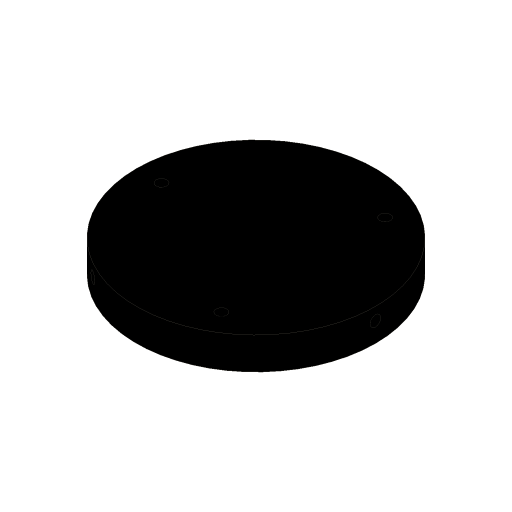
# Autodesk Inventor part: Engine bulkhead
Saved by Autodesk Inventor 2024 (Build 280153000, 153)
## iProperties
Created: 2023-12-30
Part Number: Engine bulkhead
Material: Steel AISI 1006 85 HR
Document SubType Name: Modeling
Designer: Jamie
Density: 7.872 g/cm^3
Appearance: Steel
Mass: 203.39 g
Surface Area: 95.0094 cm^2
Volume: 25.8372 cm^3
Author: Jamie
Autodesk Inventor part; units mm, degrees
ref_plane "XZ Plane" through (0, 0, 0) normal (0, 1, 0) x (-1, 0, 0)
ref_plane "XY Plane" through (0, 0, 0) normal (0, 0, 1) x (1, 0, 0)
sketch "Sketch1" plane through (0, 0, 0) normal (0, 1, 0) x (-1, 0, 0)
  circle A0 centre (0, 0) radius 33.5
  dimension "d0" = 67
  constraints: 1 centre point, 1 coincident
  measures "d0" diameter of A0
extrude "Extrusion1" add sketch "Sketch1" along normal blind 6
ref_plane "Work Plane1" through (33.5, 0, 0) normal (1, 0, 0) x (0, 1, 0)
sketch "Sketch6" plane through (33.5, 0, 0) normal (1, 0, 0) x (0, 1, 0)
  line L0 (0, -33.5) -> (0, 33.5) projected
  point P0 (0, 0)
  point P1 (2.5, 0)
  dimension "d47" = 2.5
  measures "d47" distance from line of L0 point (2.5, 0)
hole "Hole4" at (33.5, 2.5, 0) direction (-1, 0, 0) diameter 3 depth 8 tip angle 118
pattern_circular "Circular Pattern3" count 3 over 360 about axis through (0, 0, 0) along (0, 1, 0) of "Hole4"
sketch "Sketch7" plane through (0, 0, 0) normal (0, -1, 0) x (1, 0, 0)
  circle A0 centre (0, 0) radius 24.25
  circle A1 centre (0, 0) radius 33.5
  dimension "d58" = 48.5
  dimension "d59" = 67
  constraints: 2 centre point, 2 coincident
  measures "d58" diameter of A0
  measures "d59" diameter of A1
extrude "Extrusion3" add sketch "Sketch7" along normal blind 3
chamfer "Chamfer1" distance 1.5 angle 45 1 edges at (-24.25, -3, 0)
sketch "Sketch8" plane through (0, 6, 0) normal (0, 1, 0) x (1, 0, 0)
  circle A0 centre (13.25, -22.9497) radius 1.5
  circle A1 centre (0, 0) radius 33.5 construction
  line L0 (0, 0) -> (13.25, -22.9497) construction
  line L1 (0, 0) -> (33.5, 0) construction
  dimension "d65" = 3
  dimension "d66" = 26.5
  dimension "d67" = 60
  constraints: 4 end point, 1 centre point, 1 coincident, 1 horizontal, 1 horizontal alignment, 2 other
  measures "d65" diameter of A0
  measures "d66" distance of point (0, 0) L0.end
  measures "d67" angle of L1 L0
extrude "Extrusion4" cut sketch "Sketch8" against normal blind 10
pattern_circular "Circular Pattern4" count 3 over 360 about axis through (0, 0, 0) along (0, 1, 0) of "Extrusion4"
body "Solid1"
